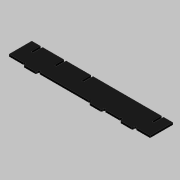
# Autodesk Inventor part: AK-C-C39-Separator
Saved by Autodesk Inventor 2016 (Build 200138000, 138)
## iProperties
Created: 2016-04-01
Part Number: AK-C-C39-Separator
Material: Generic
Document SubType Name: Modeling
Designer: admin
Density: 1 g/cm^3
Appearance: Glossy - Black
Author: admin
Autodesk Inventor part; units mm, degrees
ref_plane "YZ Plane" through (0, 0, 0) normal (1, 0, 0) x (0, 1, 0)
ref_plane "XZ Plane" through (0, 0, 0) normal (0, 1, 0) x (-1, 0, 0)
ref_plane "XY Plane" through (0, 0, 0) normal (0, 0, 1) x (1, 0, 0)
sketch "Sketch1" plane through (0, 0, 0) normal (0, 0, 1) x (1, 0, 0)
  line L0 (-57, -9.2) -> (-57, 9.2)
  line L1 (-57, 9.2) -> (-50, 9.2)
  line L2 (-50, 9.2) -> (-50, 2.2)
  line L3 (-48.25, 2.2) -> (-48.25, 9.2)
  line L4 (-48.25, 9.2) -> (-31, 9.2)
  line L5 (-31, 9.2) -> (-31, 2.2)
  line L6 (-29.25, 2.2) -> (-29.25, 9.2)
  line L7 (-29.25, 9.2) -> (-9.25, 9.2)
  line L8 (-9.25, 9.2) -> (-9.25, 2.2)
  line L9 (-7.5, 2.2) -> (-7.5, 9.2)
  line L10 (-7.5, 9.2) -> (47.75, 9.2)
  line L11 (47.75, 9.2) -> (47.75, 2.2)
  line L12 (49.5, 2.2) -> (49.5, 9.2)
  line L13 (49.5, 9.2) -> (57, 9.2)
  line L14 (57, 9.2) -> (57, -9.2)
  line L15 (57, -9.2) -> (46, -9.2)
  line L16 (44.25, -9.2) -> (44.25, -10.2)
  line L17 (43.75, -10.7) -> (34.75, -10.7)
  line L18 (34.25, -10.2) -> (34.25, -9.2)
  line L19 (32.5, -9.2) -> (21, -9.2)
  line L20 (19.25, -9.2) -> (19.25, -10.2)
  line L21 (18.75, -10.7) -> (9.75, -10.7)
  line L22 (9.25, -10.2) -> (9.25, -9.2)
  line L23 (7.5, -9.2) -> (-32, -9.2)
  line L24 (-33.75, -9.2) -> (-33.75, -10.2)
  line L25 (-34.25, -10.7) -> (-43.25, -10.7)
  line L26 (-43.75, -10.2) -> (-43.75, -9.2)
  line L27 (-45.5, -9.2) -> (-57, -9.2)
  arc A0 (-50, 2.2) -> (-48.25, 2.2) centre (-49.125, 2.2) ccw
  arc A1 (-31, 2.2) -> (-29.25, 2.2) centre (-30.125, 2.2) ccw
  arc A2 (-9.25, 2.2) -> (-7.5, 2.2) centre (-8.375, 2.2) ccw
  arc A3 (47.75, 2.2) -> (49.5, 2.2) centre (48.625, 2.2) ccw
  arc A4 (46, -9.2) -> (44.25, -9.2) centre (45.125, -9.2) ccw
  arc A5 (34.25, -9.2) -> (32.5, -9.2) centre (33.375, -9.2) ccw
  arc A6 (21, -9.2) -> (19.25, -9.2) centre (20.125, -9.2) ccw
  arc A7 (9.25, -9.2) -> (7.5, -9.2) centre (8.375, -9.2) ccw
  arc A8 (-32, -9.2) -> (-33.75, -9.2) centre (-32.875, -9.2) ccw
  arc A9 (-43.75, -9.2) -> (-45.5, -9.2) centre (-44.625, -9.2) ccw
  line L28 (0, 7.1627) -> (0, -7.1627) construction
  line L29 (-57.5, 8.9716) -> (-57.5, -9.2178) construction
  line L30 (57.5, 8.8825) -> (57.5, -9.2178) construction
  line L31 (-43.75, -10.2) -> (-43.25, -10.7)
  line L32 (-34.25, -10.7) -> (-33.75, -10.2)
  line L33 (9.25, -10.2) -> (9.75, -10.7)
  line L34 (18.75, -10.7) -> (19.25, -10.2)
  line L35 (34.25, -10.2) -> (34.75, -10.7)
  line L36 (43.75, -10.7) -> (44.25, -10.2)
  point P0 (0, 0)
  point P1 (0, 0)
  point P2 (57, 0)
  dimension "d2" = 1.75
  dimension "d3" = 7
  dimension "d7" = 1.5
  dimension "d11" = 43
  dimension "d12" = 15
  dimension "d15" = 115
  dimension "d16" = 0.5
  dimension "d17" = 0.5
  dimension "d18" = 13.75
  dimension "d19" = 13.25
  dimension "d20" = 4.5
  dimension "d21" = 2.75
  dimension "d22" = 20
  dimension "d23" = 57
  dimension "d24" = 18.4
  dimension "d25" = 135
  dimension "d26" = 0.5
  dimension "d27" = 10
  dimension "d28" = 10
  dimension "d29" = 10
  constraints: 74 end point, 21 perpendicular, 20 point on circle, 19 point on line, 14 tangent, 10 centre point, 9 equal radius, 7 vertical, 4 horizontal alignment, 4 parallel, 2 collinear, 2 midpoint, 1 coincident, 1 horizontal, 1 other
  measures "d2" diameter of A9
  measures "d3" distance from line of A0.centre L1
  measures "d7" distance between parallel lines of L23 L25
  measures "d11" distance between parallel lines of L22 L24
  measures "d12" distance between parallel lines of L18 L20
  measures "d15" distance between parallel lines of L30 L29
  measures "d16" distance between parallel lines of L29 L0
  measures "d17" distance between parallel lines of L30 L14
  measures "d18" distance between parallel lines of L26 L29
  measures "d19" distance between parallel lines of L30 L16
  measures "d20" distance between parallel lines of L26 L3
  measures "d21" distance between parallel lines of L24 L5
  measures "d22" distance between parallel lines of L8 L6
  measures "d23" distance between parallel lines of L11 L8
  measures "d24" distance between parallel lines of L15 L13
  measures "d25" angle of L25 L31
  measures "d26" distance from line of L26.start L25
  measures "d27" distance between parallel lines of L16 L18
  measures "d28" distance between parallel lines of L20 L22
  measures "d29" distance between parallel lines of L24 L26
extrude "Extrusion1" add sketch "Sketch1" along normal blind 1.6
body "Solid1"
